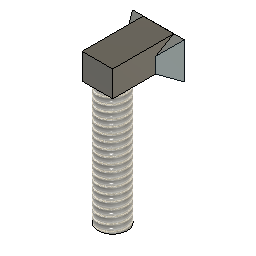
tof_rod (Autodesk Fusion 360 design; units mm, degrees)
Autodesk Fusion 360 part; units mm, degrees
sketch "Sketch1" plane through (0, 0, 0) normal (0, 0, 1) x (1, 0, 0)
  circle A0 centre (0, 0) radius 4.75
  dimension "d1" = 9.5
  constraint coincident A0.centre origin
  measures "d1" diameter of A0
extrude "Extrude1" add sketch "Sketch1" along normal blind 40
sketch "Sketch2" plane through (0, 0, 0) normal (0, 1, 0) x (1, 0, 0)
sketch "Sketch3" plane through (0, 0, 40) normal (0, 0, 1) x (-1, 0, 0)
  circle A0 centre (0, 0) radius 4.75
  line L0 (5, -5) -> (-5, -5)
  line L1 (-5, -5) -> (-5, 5)
  line L2 (-5, 5) -> (5, 5)
  line L3 (5, 5) -> (5, -5)
  line L4 (5, -5) -> (-5, 5) construction
  line L5 (-5, -5) -> (5, 5) construction
  constraint horizontal L0
  constraint perpendicular L0 L1
  constraint parallel L0 L2
  constraint parallel L1 L3
  constraint coincident L4 A0.centre
  constraint coincident L5 A0.centre
  constraint coincident A0.centre origin
extrude "Extrude2" add sketch "Sketch3" along normal blind 5 contours A0 | L0 L1 L2 L3
extrude "Extrude3" add 1 faces at (-1.6667, 5, 41.6667) along direction (0, 1, 0) blind 4
extrude "Extrude4" add 1 faces at (-1.6667, 9, 41.6667) along direction (0, 1, 0) blind 6 draft 30
sketch "Sketch4" plane through (-0.1471, 0.0849, 0) normal (0.866025, -0.5, 0) x (0.5, 0.866025, 0)
  line L0 (17.2224, 36.5359) -> (17.2224, 48.4641)
  line L1 (17.2224, 48.4641) -> (10.2942, 45)
  line L2 (10.2942, 45) -> (10.2942, 40)
  line L3 (10.2942, 40) -> (17.2224, 36.5359)
extrude "Extrude5" add 1 faces at (1.6667, 4.3333, 45) along direction (0, 0, 1) blind 3.442
extrude "Extrude6" add 1 faces at (-1.6667, 9, 46.1473) along direction (0, 1, 0) blind 6
thread "Thread4" "ACME Screw Threads 3/8 0.3750 0.3750 4G" major diameter 9.4615 minor diameter 7.0764 pitch 2.1167 angle 29 resizes the face on face at (4.7441, -0.2368, 26.6667)
